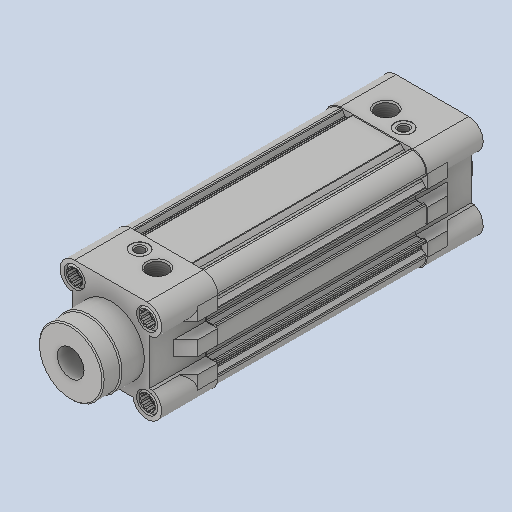
# Autodesk Inventor part: 163321 DNC-32-50---(ZR)_CPY
Saved by Autodesk Inventor 2023 (Build 270158000, 158)
## iProperties
Created: 2023-04-07
Part Number: 163321 DNC-32-50---(ZR)_CPY
Material: Generic
Catalog Web Link: www.cadenas.de
Description: DNC-(ZR)-Standard cylinder
Vendor: FESTO
Document SubType Name: Modeling
Designer: Lenovo
Manufacturer: FESTO
Mass: 206.257 g
Surface Area: 617.501 cm^2
Volume: 206.257 cm^3
Density: 1 g/cm^3
Appearance: PSOLRGB-175-175-175
Category: PARTsolutions
Company: FESTO
Title: DNC-32-50---(ZR)
Author: Cadenas PARTsolutions
Comments: Standard cylinder
PSOL_IDENT_0: {$CADENAS_DATA/23d-libs/festo/parts/d/dnc/parts/dnc_zyl.prj},223 {VTYP=3D},{NB=163321 DNC-32-50---(Z
PSOL_IDENT_1: R)},{LINA=DNC-32-50---(ZR)},{NN=DNC-(ZR)},{DATE=06.03.2020 08:57:36},{GEOMDATE=06.03.2020 08:57:36},
PSOL_IDENT_2: {VERSION=},{LINEID=10},{WBVAR=TNR,HUB,C180,Q,S2,TT,EL},{WBNUMERIC=HUB,C180,Q,S2,TT,EL}  {NB=163321 D
PSOL_IDENT_3: NC-32-50---(ZR)},{LINA=DNC-32-50---(ZR)},{KT=DUMMY},{TNR=163321},{TYP=DNC},{KDM=32},{T1=5.500},{HUB=
PSOL_IDENT_4: 50},{C180=0},{Q=0},{S2=1},{TT=0},{TTT=},{EL=0},{ZZ=0},{B=30.000},{D2=12.000},{B1=10.000},{D5=32.500}
PSOL_IDENT_5: ,{D7=M6},{D7N=6.000},{D7K=4.917},{E=45.500},{EE=G1/8},{EEN=9.728},{EEK=8.566},{EET=11.000},{J3=5.200
PSOL_IDENT_6: },{J4=6},{J5=44.500},{L2=41.600},{L3=62.800},{L4=4.000},{L5=25.100},{L6=16.000},{L7=3.300},{L8=10.00
PSOL_IDENT_7: 0},{VD=18.000},{WH=26.000},{ZB=120.000},{NA=13.700},{RE=6.000},{VL2=22.000},{C180T=},{QT=},{QN=0},{S
PSOL_IDENT_8: 2T=},{S2N=1},{ZM=97},{A1=35.000},{A2=500.000},{K1=M10},{ELT=},{ELD=13.000},{ELAV=13.900},{ELAH=12.00
PSOL_IDENT_9: 0},{ELH=10.000},{ELD2=3.000},{ELD3=1.500},{ELT1=2.000},{ELB1=6.000},{H1=57.500},{H10=7.000},{H11=0.0
PSOL_IDENT_10: 00},{MASSBASIC=0.517},{MASSHUB=0.030},{B10=6.500},{B11=7.000},{B12=10.000},{B13=11.500},{B14=2.100},
PSOL_IDENT_11: {B15=5.450},{L20=9.000},{L21=1.000},{B1ZNCM=30.000},{T2=21.000},{D100=9.500},{D101=9.000},{ANG=40.00
PSOL_IDENT_12: 0},{D102=7.400},{SW100=6.000},{L13=4.000},{V1=1.000}
NB: 163321 DNC-32-50---(ZR)
NN: DNC-(ZR)
NT: Standard cylinder
NBSYN: $TNR. $TYP.-$KDM.-$HUB.$C180T.$QT.$S2T.$TTT.$ELT.---(ZR)
LINA: DNC-32-50---(ZR)
CATALOG: Festo
TNR: 163321
TYP: DNC
KDM: 32
T1: 5.5
HUB: 50
C180: -
Q: rund
S2: normal
TT: -
EL: -
B: 30
D2: 12
B1: 10
D5: 32.5
D7: M6
D7N: 6
D7K: 4.917
E: 45.5
EE: G1/8
EEN: 9.728
EEK: 8.566
EET: 11
J3: 5.2
J4: 6
J5: 44.5
L2: 41.6
L3: 62.8
L4: 4
L5: 25.1
L6: 16
L7: 3.3
L8: 10
VD: 18
WH: 26
ZB: 120
NA: 13.7
RE: 6
VL2: 22
A1: 35
A2: 500
K1: M10
ELD: 13
ELAV: 13.9
ELAH: 12
ELH: 10
ELD2: 3
ELD3: 1.5
ELT1: 2
ELB1: 6
H1: 57.5
H10: 7
H11: 0
MASSBASIC: 0.517
MASSHUB: 0.03
B10: 6.5
B11: 7
B12: 10
B13: 11.5
B14: 2.1
B15: 5.45
L20: 9
L21: 1
B1ZNCM: 30
T2: 21
D100: 9.5
D101: 9
ANG: 40
D102: 7.4
SW100: 6
L13: 4
V1: 1
SUPPLIER: FESTO
ARTICLENO: 163321 DNC-32-50---(ZR)
BOMINFO: DNC-32-50---(ZR)
CREATOR: CADENAS GmbH
Autodesk Inventor part; units mm, degrees
sketch "Skizze_1" plane through (0, 0, 0) normal (0, 0, 1) x (1, 0, 0)
  arc A0 (-17.3, -9.8354) -> (-9.8354, -17.3) centre (-16.25, -16.25) ccw
  line L0 (-9.8354, -17.3) -> (9.8354, -17.3)
  arc A1 (9.8354, -17.3) -> (17.3, -9.8354) centre (16.25, -16.25) ccw
  line L1 (17.3, -9.8354) -> (17.3, 9.8354)
  arc A2 (17.3, 9.8354) -> (16.25, 22.75) centre (16.25, 16.25) ccw
  line L2 (16.25, 22.75) -> (-16.25, 22.75)
  arc A3 (-16.25, 22.75) -> (-17.3, 9.8354) centre (-16.25, 16.25) ccw
  line L3 (-17.3, 9.8354) -> (-17.3, -9.8354)
  constraints: 8 end point, 8 point on circle, 4 centre point
extrude "Extrusion1" add sketch "Skizze_1" against normal blind 25.1
sketch "Sketch_3" plane through (0, 0, 0) normal (1, 0, 0) x (0, 1, 0)
  line L0 (-17.3, -10.65) -> (-22.75, -16.1)
  line L1 (-22.75, -16.1) -> (-22.75, -25.1)
  line L2 (-22.75, -25.1) -> (-17.3, -25.1)
  line L3 (-17.3, -25.1) -> (-17.3, -10.65)
  constraints: 8 end point
extrude "Extrusion2" add sketch "Sketch_3" along normal mid plane 32.5
sketch "Sketch_4" plane through (0, 0, 0) normal (0, 1, 0) x (-1, 0, 0)
  line L0 (-17.3, -10.65) -> (-22.75, -16.1)
  line L1 (-22.75, -16.1) -> (-22.75, -25.1)
  line L2 (-22.75, -25.1) -> (-17.3, -25.1)
  line L3 (-17.3, -25.1) -> (-17.3, -10.65)
  constraints: 8 end point
extrude "Extrusion3" add sketch "Sketch_4" along normal mid plane 32.5
sketch "Sketch_5" plane through (0, 0, 0) normal (0, 1, 0) x (-1, 0, 0)
  line L0 (22.75, -16.1) -> (17.3, -10.65)
  line L1 (17.3, -10.65) -> (17.3, -25.1)
  line L2 (17.3, -25.1) -> (22.75, -25.1)
  line L3 (22.75, -25.1) -> (22.75, -16.1)
  constraints: 8 end point
extrude "Extrusion4" add sketch "Sketch_5" along normal mid plane 32.5
sketch "Sketch_9" plane through (0, 0, 0) normal (0, 0, 1) x (1, 0, 0)
  line L0 (-27.75, 10.25) -> (-27.75, -27.75)
  line L1 (-27.75, -27.75) -> (27.75, -27.75)
  line L2 (27.75, -27.75) -> (27.75, 10.25)
  line L3 (27.75, 10.25) -> (17.3, 10.25)
  line L4 (17.3, 10.25) -> (17.3, 3.25)
  line L5 (17.3, 3.25) -> (25.75, 3.25)
  line L6 (25.75, 3.25) -> (25.75, -3.25)
  line L7 (25.75, -3.25) -> (17.3, -3.25)
  line L8 (17.3, -3.25) -> (17.3, -10.25)
  line L9 (17.3, -10.25) -> (25.75, -10.25)
  line L10 (25.75, -10.25) -> (25.75, -25.75)
  line L11 (25.75, -25.75) -> (10.25, -25.75)
  line L12 (10.25, -25.75) -> (10.25, -17.3)
  line L13 (10.25, -17.3) -> (3.25, -17.3)
  line L14 (3.25, -17.3) -> (3.25, -25.75)
  line L15 (3.25, -25.75) -> (-3.25, -25.75)
  line L16 (-3.25, -25.75) -> (-3.25, -17.3)
  line L17 (-3.25, -17.3) -> (-10.25, -17.3)
  line L18 (-10.25, -17.3) -> (-10.25, -25.75)
  line L19 (-10.25, -25.75) -> (-25.75, -25.75)
  line L20 (-25.75, -25.75) -> (-25.75, -10.25)
  line L21 (-25.75, -10.25) -> (-17.3, -10.25)
  line L22 (-17.3, -10.25) -> (-17.3, -3.25)
  line L23 (-17.3, -3.25) -> (-25.75, -3.25)
  line L24 (-25.75, -3.25) -> (-25.75, 3.25)
  line L25 (-25.75, 3.25) -> (-17.3, 3.25)
  line L26 (-17.3, 3.25) -> (-17.3, 10.25)
  line L27 (-17.3, 10.25) -> (-27.75, 10.25)
  constraints: 56 end point
extrude "Extrusion5" cut sketch "Sketch_9" against normal blind 25.1
sketch "Skizze_2" plane through (0, 0, -25.1) normal (0, 0, 1) x (1, 0, 0)
  arc A0 (-22.25, -16.25) -> (-16.25, -22.25) centre (-16.25, -16.25) ccw
  line L0 (-16.25, -22.25) -> (-15.4099, -22.25)
  arc A1 (-15.4099, -22.25) -> (-15.0635, -22.05) centre (-15.4099, -21.85) ccw
  line L1 (-15.0635, -22.05) -> (-14.082, -20.35)
  arc A2 (-13.7356, -20.15) -> (-14.082, -20.35) centre (-13.7356, -20.55) ccw
  line L2 (-13.7356, -20.15) -> (-13.4713, -20.15)
  arc A3 (-12.4107, -20.5893) -> (-13.4713, -20.15) centre (-13.4713, -21.65) ccw
  line L3 (-12.4107, -20.5893) -> (-10.8672, -22.1328)
  arc A4 (-10.8672, -22.1328) -> (-10.5843, -22.25) centre (-10.5843, -21.85) ccw
  line L4 (-10.5843, -22.25) -> (-9.85, -22.25)
  arc A5 (-9.85, -22.25) -> (-9.45, -21.85) centre (-9.85, -21.85) ccw
  line L5 (-9.45, -21.85) -> (-9.45, -21.15)
  arc A6 (-9.45, -21.15) -> (-9.65, -20.95) centre (-9.65, -21.15) ccw
  line L6 (-9.65, -20.95) -> (-9.9, -20.95)
  arc A7 (-10.1, -20.75) -> (-9.9, -20.95) centre (-9.9, -20.75) ccw
  line L7 (-10.1, -20.75) -> (-10.1, -18.05)
  arc A8 (-9.7, -17.65) -> (-10.1, -18.05) centre (-9.7, -18.05) ccw
  line L8 (-9.7, -17.65) -> (-4, -17.65)
  arc A9 (-3.6, -18.05) -> (-4, -17.65) centre (-4, -18.05) ccw
  line L9 (-3.6, -18.05) -> (-3.6, -20.75)
  arc A10 (-3.8, -20.95) -> (-3.6, -20.75) centre (-3.8, -20.75) ccw
  line L10 (-3.8, -20.95) -> (-4.05, -20.95)
  arc A11 (-4.05, -20.95) -> (-4.25, -21.15) centre (-4.05, -21.15) ccw
  line L11 (-4.25, -21.15) -> (-4.25, -21.85)
  arc A12 (-4.25, -21.85) -> (-3.85, -22.25) centre (-3.85, -21.85) ccw
  line L12 (-3.85, -22.25) -> (3.85, -22.25)
  arc A13 (3.85, -22.25) -> (4.25, -21.85) centre (3.85, -21.85) ccw
  line L13 (4.25, -21.85) -> (4.25, -21.15)
  arc A14 (4.25, -21.15) -> (4.05, -20.95) centre (4.05, -21.15) ccw
  line L14 (4.05, -20.95) -> (3.8, -20.95)
  arc A15 (3.6, -20.75) -> (3.8, -20.95) centre (3.8, -20.75) ccw
  line L15 (3.6, -20.75) -> (3.6, -18.05)
  arc A16 (4, -17.65) -> (3.6, -18.05) centre (4, -18.05) ccw
  line L16 (4, -17.65) -> (9.7, -17.65)
  arc A17 (10.1, -18.05) -> (9.7, -17.65) centre (9.7, -18.05) ccw
  line L17 (10.1, -18.05) -> (10.1, -20.75)
  arc A18 (9.9, -20.95) -> (10.1, -20.75) centre (9.9, -20.75) ccw
  line L18 (9.9, -20.95) -> (9.65, -20.95)
  arc A19 (9.65, -20.95) -> (9.45, -21.15) centre (9.65, -21.15) ccw
  line L19 (9.45, -21.15) -> (9.45, -21.85)
  arc A20 (9.45, -21.85) -> (9.85, -22.25) centre (9.85, -21.85) ccw
  line L20 (9.85, -22.25) -> (10.5843, -22.25)
  arc A21 (10.5843, -22.25) -> (10.8672, -22.1328) centre (10.5843, -21.85) ccw
  line L21 (10.8672, -22.1328) -> (12.4107, -20.5893)
  arc A22 (13.4713, -20.15) -> (12.4107, -20.5893) centre (13.4713, -21.65) ccw
  line L22 (13.4713, -20.15) -> (13.7356, -20.15)
  arc A23 (14.082, -20.35) -> (13.7356, -20.15) centre (13.7356, -20.55) ccw
  line L23 (14.082, -20.35) -> (15.0635, -22.05)
  arc A24 (15.0635, -22.05) -> (15.4099, -22.25) centre (15.4099, -21.85) ccw
  line L24 (15.4099, -22.25) -> (16.25, -22.25)
  arc A25 (16.25, -22.25) -> (22.25, -16.25) centre (16.25, -16.25) ccw
  line L25 (22.25, -16.25) -> (22.25, -15.4099)
  arc A26 (22.25, -15.4099) -> (22.05, -15.0635) centre (21.85, -15.4099) ccw
  line L26 (22.05, -15.0635) -> (20.35, -14.082)
  arc A27 (20.15, -13.7356) -> (20.35, -14.082) centre (20.55, -13.7356) ccw
  line L27 (20.15, -13.7356) -> (20.15, -13.4713)
  arc A28 (20.5893, -12.4107) -> (20.15, -13.4713) centre (21.65, -13.4713) ccw
  line L28 (20.5893, -12.4107) -> (22.1328, -10.8672)
  arc A29 (22.1328, -10.8672) -> (22.25, -10.5843) centre (21.85, -10.5843) ccw
  line L29 (22.25, -10.5843) -> (22.25, -9.85)
  arc A30 (22.25, -9.85) -> (21.85, -9.45) centre (21.85, -9.85) ccw
  line L30 (21.85, -9.45) -> (21.15, -9.45)
  arc A31 (21.15, -9.45) -> (20.95, -9.65) centre (21.15, -9.65) ccw
  line L31 (20.95, -9.65) -> (20.95, -9.9)
  arc A32 (20.75, -10.1) -> (20.95, -9.9) centre (20.75, -9.9) ccw
  line L32 (20.75, -10.1) -> (18.05, -10.1)
  arc A33 (17.65, -9.7) -> (18.05, -10.1) centre (18.05, -9.7) ccw
  line L33 (17.65, -9.7) -> (17.65, -4)
  arc A34 (18.05, -3.6) -> (17.65, -4) centre (18.05, -4) ccw
  line L34 (18.05, -3.6) -> (20.75, -3.6)
  arc A35 (20.95, -3.8) -> (20.75, -3.6) centre (20.75, -3.8) ccw
  line L35 (20.95, -3.8) -> (20.95, -4.05)
  arc A36 (20.95, -4.05) -> (21.15, -4.25) centre (21.15, -4.05) ccw
  line L36 (21.15, -4.25) -> (21.85, -4.25)
  arc A37 (21.85, -4.25) -> (22.25, -3.85) centre (21.85, -3.85) ccw
  line L37 (22.25, -3.85) -> (22.25, 3.85)
  arc A38 (22.25, 3.85) -> (21.85, 4.25) centre (21.85, 3.85) ccw
  line L38 (21.85, 4.25) -> (21.15, 4.25)
  arc A39 (21.15, 4.25) -> (20.95, 4.05) centre (21.15, 4.05) ccw
  line L39 (20.95, 4.05) -> (20.95, 3.8)
  arc A40 (20.75, 3.6) -> (20.95, 3.8) centre (20.75, 3.8) ccw
  line L40 (20.75, 3.6) -> (18.05, 3.6)
  arc A41 (17.65, 4) -> (18.05, 3.6) centre (18.05, 4) ccw
  line L41 (17.65, 4) -> (17.65, 9.7)
  arc A42 (18.05, 10.1) -> (17.65, 9.7) centre (18.05, 9.7) ccw
  line L42 (18.05, 10.1) -> (20.75, 10.1)
  arc A43 (20.95, 9.9) -> (20.75, 10.1) centre (20.75, 9.9) ccw
  line L43 (20.95, 9.9) -> (20.95, 9.65)
  arc A44 (20.95, 9.65) -> (21.15, 9.45) centre (21.15, 9.65) ccw
  line L44 (21.15, 9.45) -> (21.85, 9.45)
  arc A45 (21.85, 9.45) -> (22.25, 9.85) centre (21.85, 9.85) ccw
  line L45 (22.25, 9.85) -> (22.25, 10.5843)
  arc A46 (22.25, 10.5843) -> (22.1328, 10.8672) centre (21.85, 10.5843) ccw
  line L46 (22.1328, 10.8672) -> (20.5893, 12.4107)
  arc A47 (20.15, 13.4713) -> (20.5893, 12.4107) centre (21.65, 13.4713) ccw
  line L47 (20.15, 13.4713) -> (20.15, 13.7356)
  arc A48 (20.35, 14.082) -> (20.15, 13.7356) centre (20.55, 13.7356) ccw
  line L48 (20.35, 14.082) -> (22.05, 15.0635)
  arc A49 (22.05, 15.0635) -> (22.25, 15.4099) centre (21.85, 15.4099) ccw
  line L49 (22.25, 15.4099) -> (22.25, 16.25)
  arc A50 (22.25, 16.25) -> (16.25, 22.25) centre (16.25, 16.25) ccw
  line L50 (16.25, 22.25) -> (15.4099, 22.25)
  arc A51 (15.4099, 22.25) -> (15.0635, 22.05) centre (15.4099, 21.85) ccw
  line L51 (15.0635, 22.05) -> (14.082, 20.35)
  arc A52 (13.7356, 20.15) -> (14.082, 20.35) centre (13.7356, 20.55) ccw
  line L52 (13.7356, 20.15) -> (13.4713, 20.15)
  arc A53 (12.4107, 20.5893) -> (13.4713, 20.15) centre (13.4713, 21.65) ccw
  line L53 (12.4107, 20.5893) -> (10.8672, 22.1328)
  arc A54 (10.8672, 22.1328) -> (10.5843, 22.25) centre (10.5843, 21.85) ccw
  line L54 (10.5843, 22.25) -> (-10.5843, 22.25)
  arc A55 (-10.5843, 22.25) -> (-10.8672, 22.1328) centre (-10.5843, 21.85) ccw
  line L55 (-10.8672, 22.1328) -> (-12.4107, 20.5893)
  arc A56 (-13.4713, 20.15) -> (-12.4107, 20.5893) centre (-13.4713, 21.65) ccw
  line L56 (-13.4713, 20.15) -> (-13.7356, 20.15)
  arc A57 (-14.082, 20.35) -> (-13.7356, 20.15) centre (-13.7356, 20.55) ccw
  line L57 (-14.082, 20.35) -> (-15.0635, 22.05)
  arc A58 (-15.0635, 22.05) -> (-15.4099, 22.25) centre (-15.4099, 21.85) ccw
  line L58 (-15.4099, 22.25) -> (-16.25, 22.25)
  arc A59 (-16.25, 22.25) -> (-22.25, 16.25) centre (-16.25, 16.25) ccw
  line L59 (-22.25, 16.25) -> (-22.25, 15.4099)
  arc A60 (-22.25, 15.4099) -> (-22.05, 15.0635) centre (-21.85, 15.4099) ccw
  line L60 (-22.05, 15.0635) -> (-20.35, 14.082)
  arc A61 (-20.15, 13.7356) -> (-20.35, 14.082) centre (-20.55, 13.7356) ccw
  line L61 (-20.15, 13.7356) -> (-20.15, 13.4713)
  arc A62 (-20.5893, 12.4107) -> (-20.15, 13.4713) centre (-21.65, 13.4713) ccw
  line L62 (-20.5893, 12.4107) -> (-22.1328, 10.8672)
  arc A63 (-22.1328, 10.8672) -> (-22.25, 10.5843) centre (-21.85, 10.5843) ccw
  line L63 (-22.25, 10.5843) -> (-22.25, 9.85)
  arc A64 (-22.25, 9.85) -> (-21.85, 9.45) centre (-21.85, 9.85) ccw
  line L64 (-21.85, 9.45) -> (-21.15, 9.45)
  arc A65 (-21.15, 9.45) -> (-20.95, 9.65) centre (-21.15, 9.65) ccw
  line L65 (-20.95, 9.65) -> (-20.95, 9.9)
  arc A66 (-20.75, 10.1) -> (-20.95, 9.9) centre (-20.75, 9.9) ccw
  line L66 (-20.75, 10.1) -> (-18.05, 10.1)
  arc A67 (-17.65, 9.7) -> (-18.05, 10.1) centre (-18.05, 9.7) ccw
  line L67 (-17.65, 9.7) -> (-17.65, 4)
  arc A68 (-18.05, 3.6) -> (-17.65, 4) centre (-18.05, 4) ccw
  line L68 (-18.05, 3.6) -> (-20.75, 3.6)
  arc A69 (-20.95, 3.8) -> (-20.75, 3.6) centre (-20.75, 3.8) ccw
  line L69 (-20.95, 3.8) -> (-20.95, 4.05)
  arc A70 (-20.95, 4.05) -> (-21.15, 4.25) centre (-21.15, 4.05) ccw
  line L70 (-21.15, 4.25) -> (-21.85, 4.25)
  arc A71 (-21.85, 4.25) -> (-22.25, 3.85) centre (-21.85, 3.85) ccw
  line L71 (-22.25, 3.85) -> (-22.25, -3.85)
  arc A72 (-22.25, -3.85) -> (-21.85, -4.25) centre (-21.85, -3.85) ccw
  line L72 (-21.85, -4.25) -> (-21.15, -4.25)
  arc A73 (-21.15, -4.25) -> (-20.95, -4.05) centre (-21.15, -4.05) ccw
  line L73 (-20.95, -4.05) -> (-20.95, -3.8)
  arc A74 (-20.75, -3.6) -> (-20.95, -3.8) centre (-20.75, -3.8) ccw
  line L74 (-20.75, -3.6) -> (-18.05, -3.6)
  arc A75 (-17.65, -4) -> (-18.05, -3.6) centre (-18.05, -4) ccw
  line L75 (-17.65, -4) -> (-17.65, -9.7)
  arc A76 (-18.05, -10.1) -> (-17.65, -9.7) centre (-18.05, -9.7) ccw
  line L76 (-18.05, -10.1) -> (-20.75, -10.1)
  arc A77 (-20.95, -9.9) -> (-20.75, -10.1) centre (-20.75, -9.9) ccw
  line L77 (-20.95, -9.9) -> (-20.95, -9.65)
  arc A78 (-20.95, -9.65) -> (-21.15, -9.45) centre (-21.15, -9.65) ccw
  line L78 (-21.15, -9.45) -> (-21.85, -9.45)
  arc A79 (-21.85, -9.45) -> (-22.25, -9.85) centre (-21.85, -9.85) ccw
  line L79 (-22.25, -9.85) -> (-22.25, -10.5843)
  arc A80 (-22.25, -10.5843) -> (-22.1328, -10.8672) centre (-21.85, -10.5843) ccw
  line L80 (-22.1328, -10.8672) -> (-20.5893, -12.4107)
  arc A81 (-20.15, -13.4713) -> (-20.5893, -12.4107) centre (-21.65, -13.4713) ccw
  line L81 (-20.15, -13.4713) -> (-20.15, -13.7356)
  arc A82 (-20.35, -14.082) -> (-20.15, -13.7356) centre (-20.55, -13.7356) ccw
  line L82 (-20.35, -14.082) -> (-22.05, -15.0635)
  arc A83 (-22.05, -15.0635) -> (-22.25, -15.4099) centre (-21.85, -15.4099) ccw
  line L83 (-22.25, -15.4099) -> (-22.25, -16.25)
  constraints: 168 end point, 168 point on circle, 84 centre point
extrude "Extrusion6" add sketch "Skizze_2" against normal blind 93.8
sketch "Skizze_3" plane through (0, 0, -118.9) normal (0, 0, 1) x (1, 0, 0)
  arc A0 (-17.3, -9.8354) -> (-9.8354, -17.3) centre (-16.25, -16.25) ccw
  line L0 (-9.8354, -17.3) -> (9.8354, -17.3)
  arc A1 (9.8354, -17.3) -> (17.3, -9.8354) centre (16.25, -16.25) ccw
  line L1 (17.3, -9.8354) -> (17.3, 9.8354)
  arc A2 (17.3, 9.8354) -> (16.25, 22.75) centre (16.25, 16.25) ccw
  line L2 (16.25, 22.75) -> (-16.25, 22.75)
  arc A3 (-16.25, 22.75) -> (-17.3, 9.8354) centre (-16.25, 16.25) ccw
  line L3 (-17.3, 9.8354) -> (-17.3, -9.8354)
  constraints: 8 end point, 8 point on circle, 4 centre point
extrude "Extrusion7" add sketch "Skizze_3" against normal blind 25.1
sketch "Sketch_6" plane through (0, 0, 0) normal (1, 0, 0) x (0, 1, 0)
  line L0 (-17.3, -118.9) -> (-22.75, -118.9)
  line L1 (-22.75, -118.9) -> (-22.75, -127.9)
  line L2 (-22.75, -127.9) -> (-17.3, -133.35)
  line L3 (-17.3, -133.35) -> (-17.3, -118.9)
  constraints: 8 end point
extrude "Extrusion8" add sketch "Sketch_6" along normal mid plane 32.5
sketch "Sketch_7" plane through (0, 0, 0) normal (0, 1, 0) x (-1, 0, 0)
  line L0 (-17.3, -133.35) -> (-17.3, -118.9)
  line L1 (-17.3, -118.9) -> (-22.75, -118.9)
  line L2 (-22.75, -118.9) -> (-22.75, -127.9)
  line L3 (-22.75, -127.9) -> (-17.3, -133.35)
  constraints: 8 end point
extrude "Extrusion9" add sketch "Sketch_7" along normal mid plane 32.5
sketch "Sketch_8" plane through (0, 0, 0) normal (0, 1, 0) x (-1, 0, 0)
  line L0 (22.75, -127.9) -> (22.75, -118.9)
  line L1 (22.75, -118.9) -> (17.3, -118.9)
  line L2 (17.3, -118.9) -> (17.3, -133.35)
  line L3 (17.3, -133.35) -> (22.75, -127.9)
  constraints: 8 end point
extrude "Extrusion10" add sketch "Sketch_8" along normal mid plane 32.5
sketch "Sketch_10" plane through (0, 0, -118.9) normal (0, 0, 1) x (1, 0, 0)
  line L0 (-27.75, 10.25) -> (-27.75, -27.75)
  line L1 (-27.75, -27.75) -> (27.75, -27.75)
  line L2 (27.75, -27.75) -> (27.75, 10.25)
  line L3 (27.75, 10.25) -> (17.3, 10.25)
  line L4 (17.3, 10.25) -> (17.3, 3.25)
  line L5 (17.3, 3.25) -> (25.75, 3.25)
  line L6 (25.75, 3.25) -> (25.75, -3.25)
  line L7 (25.75, -3.25) -> (17.3, -3.25)
  line L8 (17.3, -3.25) -> (17.3, -10.25)
  line L9 (17.3, -10.25) -> (25.75, -10.25)
  line L10 (25.75, -10.25) -> (25.75, -25.75)
  line L11 (25.75, -25.75) -> (10.25, -25.75)
  line L12 (10.25, -25.75) -> (10.25, -17.3)
  line L13 (10.25, -17.3) -> (3.25, -17.3)
  line L14 (3.25, -17.3) -> (3.25, -25.75)
  line L15 (3.25, -25.75) -> (-3.25, -25.75)
  line L16 (-3.25, -25.75) -> (-3.25, -17.3)
  line L17 (-3.25, -17.3) -> (-10.25, -17.3)
  line L18 (-10.25, -17.3) -> (-10.25, -25.75)
  line L19 (-10.25, -25.75) -> (-25.75, -25.75)
  line L20 (-25.75, -25.75) -> (-25.75, -10.25)
  line L21 (-25.75, -10.25) -> (-17.3, -10.25)
  line L22 (-17.3, -10.25) -> (-17.3, -3.25)
  line L23 (-17.3, -3.25) -> (-25.75, -3.25)
  line L24 (-25.75, -3.25) -> (-25.75, 3.25)
  line L25 (-25.75, 3.25) -> (-17.3, 3.25)
  line L26 (-17.3, 3.25) -> (-17.3, 10.25)
  line L27 (-17.3, 10.25) -> (-27.75, 10.25)
  constraints: 56 end point
extrude "Extrusion11" cut sketch "Sketch_10" against normal blind 25.1
sketch "Sketch_14" plane through (16.25, 0, 0) normal (1, 0, 0) x (0, 0, -1)
  line L0 (21, 16.25) -> (0, 16.25)
  line L1 (0, 16.25) -> (0, 21)
  line L2 (0, 21) -> (21, 21)
  line L3 (21, 21) -> (21, 16.25)
  line L4 (21, 16.25) -> (0, 16.25)
  constraints: 10 end point
revolve "Revolution1" cut sketch "Sketch_14" angle 360 about axis through (16.25, 16.25, -21) along (0, 0, -1)
pattern_linear "Rectangular Pattern1" count 2 spacing 32.5 along (-1, 0, 0) count 2 spacing 32.5 along (0, -1, 0) of "Revolution1"
sketch "Sketch_15" plane through (16.25, 0, 0) normal (1, 0, 0) x (0, 0, -1)
  line L0 (21, 16.25) -> (0, 16.25)
  line L1 (0, 16.25) -> (0, 19.9109)
  line L2 (0, 19.9109) -> (1, 20.75)
  line L3 (1, 20.75) -> (21, 20.75)
  line L4 (21, 20.75) -> (21, 16.25)
  line L5 (21, 16.25) -> (0, 16.25)
  constraints: 12 end point
revolve "Revolution2" add sketch "Sketch_15" angle 360 about axis through (16.25, 16.25, -21) along (0, 0, -1)
pattern_linear "Rectangular Pattern2" count 2 spacing 32.5 along (-1, 0, 0) count 2 spacing 32.5 along (0, -1, 0) of "Revolution2"
sketch "Skizze_8" plane through (16.25, 0, 0) normal (1, 0, 0) x (0, 0, -1)
  line L0 (21.3333, 16.25) -> (0, 16.25)
  line L1 (0, 16.25) -> (0, 19.95)
  line L2 (0, 19.95) -> (0.4041, 19.25)
  line L3 (0.4041, 19.25) -> (5.5, 19.25)
  line L4 (5.5, 19.25) -> (6.0415, 18.7085)
  line L5 (6.0415, 18.7085) -> (19.9139, 18.7085)
  line L6 (19.9139, 18.7085) -> (21.3333, 16.25)
  line L7 (21.3333, 16.25) -> (0, 16.25)
  constraints: 16 end point
revolve "Revolution3" cut sketch "Skizze_8" angle 360 about axis through (16.25, 16.25, -21.3333) along (0, 0, -1)
thread "Thread1" size "M6x1" class "6H" standard "ISO Metric profile" length 9.9585
pattern_linear "Rectangular Pattern3" count 2 spacing 32.5 along (-1, 0, 0) count 2 spacing 32.5 along (0, -1, 0) of "Revolution3"
sketch "Sketch_19" plane through (0, 0, 0) normal (0, 0, 1) x (1, 0, 0)
  line L0 (12.7859, 16.25) -> (13.25, 15.4462)
  line L1 (13.25, 15.4462) -> (13.25, 14.5179)
  line L2 (13.25, 14.5179) -> (14.0538, 14.0538)
  line L3 (14.0538, 14.0538) -> (14.5179, 13.25)
  line L4 (14.5179, 13.25) -> (15.4462, 13.25)
  line L5 (15.4462, 13.25) -> (16.25, 12.7859)
  line L6 (16.25, 12.7859) -> (17.0538, 13.25)
  line L7 (17.0538, 13.25) -> (17.9821, 13.25)
  line L8 (17.9821, 13.25) -> (18.4462, 14.0538)
  line L9 (18.4462, 14.0538) -> (19.25, 14.5179)
  line L10 (19.25, 14.5179) -> (19.25, 15.4462)
  line L11 (19.25, 15.4462) -> (19.7141, 16.25)
  line L12 (19.7141, 16.25) -> (19.25, 17.0538)
  line L13 (19.25, 17.0538) -> (19.25, 17.9821)
  line L14 (19.25, 17.9821) -> (18.4462, 18.4462)
  line L15 (18.4462, 18.4462) -> (17.9821, 19.25)
  line L16 (17.9821, 19.25) -> (17.0538, 19.25)
  line L17 (17.0538, 19.25) -> (16.25, 19.7141)
  line L18 (16.25, 19.7141) -> (15.4462, 19.25)
  line L19 (15.4462, 19.25) -> (14.5179, 19.25)
  line L20 (14.5179, 19.25) -> (14.0538, 18.4462)
  line L21 (14.0538, 18.4462) -> (13.25, 17.9821)
  line L22 (13.25, 17.9821) -> (13.25, 17.0538)
  line L23 (13.25, 17.0538) -> (12.7859, 16.25)
  constraints: 48 end point
extrude "Extrusion12" cut sketch "Sketch_19" against normal blind 4
pattern_linear "Rectangular Pattern4" count 2 spacing 32.5 along (-1, 0, 0) count 2 spacing 32.5 along (0, -1, 0) of "Extrusion12"
sketch "Sketch16" plane through (0, 0, -144) normal (0, 0, -1) x (-1, 0, 0)
  point P0 (-16.25, 16.25)
hole "Hole1" at (16.25, 16.25, -144) direction (0, 0, 1) diameter 9.5 depth 21
pattern_linear "Rectangular Pattern5" count 2 spacing 32.5 along (-1, 0, 0) count 2 spacing 32.5 along (0, -1, 0) of "Hole1"
sketch "Sketch_23" plane through (16.25, 0, 0) normal (1, 0, 0) x (0, 0, -1)
  line L0 (144, 16.25) -> (123, 16.25)
  line L1 (123, 16.25) -> (123, 20.75)
  line L2 (123, 20.75) -> (143, 20.75)
  line L3 (143, 20.75) -> (144, 19.9109)
  line L4 (144, 19.9109) -> (144, 16.25)
  line L5 (144, 16.25) -> (123, 16.25)
  constraints: 12 end point
revolve "Revolution4" add sketch "Sketch_23" angle 360 about axis through (16.25, 16.25, -144) along (0, 0, -1)
pattern_linear "Rectangular Pattern6" count 2 spacing 32.5 along (-1, 0, 0) count 2 spacing 32.5 along (0, -1, 0) of "Revolution4"
sketch "Sketch_25" plane through (16.25, 0, 0) normal (1, 0, 0) x (0, 0, -1)
  line L0 (144, 16.25) -> (122.6667, 16.25)
  line L1 (122.6667, 16.25) -> (124.0861, 18.7085)
  line L2 (124.0861, 18.7085) -> (137.9585, 18.7085)
  line L3 (137.9585, 18.7085) -> (138.5, 19.25)
  line L4 (138.5, 19.25) -> (143.5959, 19.25)
  line L5 (143.5959, 19.25) -> (144, 19.95)
  line L6 (144, 19.95) -> (144, 16.25)
  line L7 (144, 16.25) -> (122.6667, 16.25)
  constraints: 16 end point
revolve "Revolution5" cut sketch "Sketch_25" angle 360 about axis through (16.25, 16.25, -144) along (0, 0, -1)
thread "Thread2" size "M6x1" class "6H" standard "ISO Metric profile" length 9.9585
pattern_linear "Rectangular Pattern7" count 2 spacing 32.5 along (-1, 0, 0) count 2 spacing 32.5 along (0, -1, 0) of "Revolution5"
sketch "Sketch_27" plane through (0, 0, -144) normal (0, 0, 1) x (1, 0, 0)
  line L0 (12.7859, 16.25) -> (13.25, 15.4462)
  line L1 (13.25, 15.4462) -> (13.25, 14.5179)
  line L2 (13.25, 14.5179) -> (14.0538, 14.0538)
  line L3 (14.0538, 14.0538) -> (14.5179, 13.25)
  line L4 (14.5179, 13.25) -> (15.4462, 13.25)
  line L5 (15.4462, 13.25) -> (16.25, 12.7859)
  line L6 (16.25, 12.7859) -> (17.0538, 13.25)
  line L7 (17.0538, 13.25) -> (17.9821, 13.25)
  line L8 (17.9821, 13.25) -> (18.4462, 14.0538)
  line L9 (18.4462, 14.0538) -> (19.25, 14.5179)
  line L10 (19.25, 14.5179) -> (19.25, 15.4462)
  line L11 (19.25, 15.4462) -> (19.7141, 16.25)
  line L12 (19.7141, 16.25) -> (19.25, 17.0538)
  line L13 (19.25, 17.0538) -> (19.25, 17.9821)
  line L14 (19.25, 17.9821) -> (18.4462, 18.4462)
  line L15 (18.4462, 18.4462) -> (17.9821, 19.25)
  line L16 (17.9821, 19.25) -> (17.0538, 19.25)
  line L17 (17.0538, 19.25) -> (16.25, 19.7141)
  line L18 (16.25, 19.7141) -> (15.4462, 19.25)
  line L19 (15.4462, 19.25) -> (14.5179, 19.25)
  line L20 (14.5179, 19.25) -> (14.0538, 18.4462)
  line L21 (14.0538, 18.4462) -> (13.25, 17.9821)
  line L22 (13.25, 17.9821) -> (13.25, 17.0538)
  line L23 (13.25, 17.0538) -> (12.7859, 16.25)
  constraints: 48 end point
extrude "Extrusion13" cut sketch "Sketch_27" along normal blind 4
pattern_linear "Rectangular Pattern8" count 2 spacing 32.5 along (-1, 0, 0) count 2 spacing 32.5 along (0, -1, 0) of "Extrusion13"
sketch "Skizze_13" plane through (0, 0, 0) normal (1, 0, 0) x (0, 1, 0)
  line L0 (0, 0) -> (0, 18)
  line L1 (0, 18) -> (14, 18)
  line L2 (14, 18) -> (14.5, 17.5)
  line L3 (14.5, 17.5) -> (14.5, 10.5)
  line L4 (14.5, 10.5) -> (15, 10)
  line L5 (15, 10) -> (15, 0)
  line L6 (15, 0) -> (0, 0)
  line L7 (0, 0) -> (0, 18)
  constraints: 16 end point
revolve "Revolution6" add sketch "Skizze_13" angle 360 about axis through (0, 0, 0) along (0, 0, -1)
sketch "Sketch21" plane through (-16.25, 22.75, 0) normal (0, 1, 0) x (1, 0, 0)
  point P0 (21.45, 15.6)
hole "Hole2" at (5.2, 22.75, -15.6) direction (0, -1, 0) diameter 8.566 depth 11 countersink diameter 9.728 countersink angle 90 thread size "G9.728x0.907" designation "G 1/8" standard "ISO Pipe Threads"
sketch "Sketch_49" plane through (0, 0, -18.9) normal (0, 0, 1) x (1, 0, 0)
  line L0 (-6, 20.1167) -> (-6, 23.65)
  line L1 (-6, 23.65) -> (-2, 23.65)
  line L2 (-2, 23.65) -> (-2, 22.15)
  line L3 (-2, 22.15) -> (-2.0882, 22.65)
  line L4 (-2.0882, 22.65) -> (-3.5, 22.65)
  line L5 (-3.5, 22.65) -> (-3.933, 22.217)
  line L6 (-3.933, 22.217) -> (-3.933, 19.6167)
  line L7 (-3.933, 19.6167) -> (-4.433, 20.1167)
  line L8 (-4.433, 20.1167) -> (-6, 20.1167)
  line L9 (-6, 20.1167) -> (-6, 23.65)
  constraints: 20 end point
revolve "Revolution7" cut sketch "Sketch_49" angle 360 about axis through (-6, 20.1167, -18.9) along (0, -1, 0)
thread "Thread3" size "M5x0.8" class "6H" standard "ISO Metric profile" full length
sketch "Sketch_50" plane through (-6, 20.1167, -18.9) normal (0, 1, 0) x (1, 0, 0)
  line L0 (-0.25, -2) -> (0.25, -2)
  line L1 (0.25, -2) -> (0.25, 2)
  line L2 (0.25, 2) -> (-0.25, 2)
  line L3 (-0.25, 2) -> (-0.25, -2)
  constraints: 8 end point
extrude "Extrusion14" cut sketch "Sketch_50" against normal blind 1.5
sketch "Sketch24" plane through (-16.25, 22.75, -118.9) normal (0, 1, 0) x (1, 0, 0)
  point P0 (11.05, 9.5)
hole "Hole3" at (-5.2, 22.75, -128.4) direction (0, -1, 0) diameter 8.566 depth 11 countersink diameter 9.728 countersink angle 90 thread size "G9.728x0.907" designation "G 1/8" standard "ISO Pipe Threads"
sketch "Sketch_51" plane through (0, 0, -125.1) normal (0, 0, 1) x (1, 0, 0)
  line L0 (6, 23.65) -> (6, 20.1167)
  line L1 (6, 20.1167) -> (4.433, 20.1167)
  line L2 (4.433, 20.1167) -> (3.933, 19.6167)
  line L3 (3.933, 19.6167) -> (3.933, 22.217)
  line L4 (3.933, 22.217) -> (3.5, 22.65)
  line L5 (3.5, 22.65) -> (2.0882, 22.65)
  line L6 (2.0882, 22.65) -> (2, 22.15)
  line L7 (2, 22.15) -> (2, 23.65)
  line L8 (2, 23.65) -> (6, 23.65)
  line L9 (6, 23.65) -> (6, 20.1167)
  constraints: 20 end point
revolve "Revolution8" cut sketch "Sketch_51" angle 360 about axis through (6, 23.65, -125.1) along (0, 1, 0)
thread "Thread4" size "M5x0.8" class "6H" standard "ISO Metric profile" full length
sketch "Sketch_52" plane through (6, 20.1167, -125.1) normal (0, 1, 0) x (-1, 0, 0)
  line L0 (-0.25, -2) -> (0.25, -2)
  line L1 (0.25, -2) -> (0.25, 2)
  line L2 (0.25, 2) -> (-0.25, 2)
  line L3 (-0.25, 2) -> (-0.25, -2)
  constraints: 8 end point
extrude "Extrusion15" cut sketch "Sketch_52" against normal blind 1.5
sketch "Skizze_17" plane through (0, 0, 0) normal (1, 0, 0) x (0, 1, 0)
  line L0 (0, -148) -> (0, -144)
  line L1 (0, -144) -> (15, -144)
  line L2 (15, -144) -> (15, -147)
  line L3 (15, -147) -> (14, -148)
  line L4 (14, -148) -> (0, -148)
  line L5 (0, -148) -> (0, -144)
  constraints: 12 end point
revolve "Revolution9" add sketch "Skizze_17" angle 360 about axis through (0, 0, -148) along (0, 0, -1)
sketch "Sketch28" plane through (0, 0, 18) normal (0, 0, 1) x (1, 0, 0)
  point P0 (0, 0)
hole "Hole4" at (0, 0, 18) direction (0, 0, -1) diameter 12 depth 64.0333
sketch "Skizze_19" plane through (0, 0, 0) normal (1, 0, 0) x (0, 1, 0)
  line L0 (0, -97) -> (0, -38)
  line L1 (0, -38) -> (3, -38)
  line L2 (3, -38) -> (3, -41)
  line L3 (3, -41) -> (16, -41)
  line L4 (16, -41) -> (16, -97)
  line L5 (16, -97) -> (0, -97)
  line L6 (0, -97) -> (0, -38)
  constraints: 14 end point
revolve "Revolution10" cut sketch "Skizze_19" angle 360 about axis through (0, 0, -97) along (0, 0, -1)
ref_plane "CP_hinten_5_XY" through (16.25, 16.25, -144) normal (0, 0, 1) x (1, 0, 0)
ref_plane "CP_hinten_5_YZ" through (16.25, 16.25, -144) normal (1, 0, 0) x (0, 1, 0)
ref_plane "CP_hinten_5_ZX" through (16.25, 16.25, -144) normal (0, 1, 0) x (0, 0, 1)
ref_plane "CP_hinten_6_XY" through (16.25, -16.25, -144) normal (0, 0, 1) x (1, 0, 0)
ref_plane "CP_hinten_6_YZ" through (16.25, -16.25, -144) normal (1, 0, 0) x (0, 1, 0)
ref_plane "CP_hinten_6_ZX" through (16.25, -16.25, -144) normal (0, 1, 0) x (0, 0, 1)
ref_plane "CP_hinten_7_XY" through (-16.25, -16.25, -144) normal (0, 0, 1) x (1, 0, 0)
ref_plane "CP_hinten_7_YZ" through (-16.25, -16.25, -144) normal (1, 0, 0) x (0, 1, 0)
ref_plane "CP_hinten_7_ZX" through (-16.25, -16.25, -144) normal (0, 1, 0) x (0, 0, 1)
ref_plane "CP_hinten_8_XY" through (-16.25, 16.25, -144) normal (0, 0, 1) x (1, 0, 0)
ref_plane "CP_hinten_8_YZ" through (-16.25, 16.25, -144) normal (1, 0, 0) x (0, 1, 0)
ref_plane "CP_hinten_8_ZX" through (-16.25, 16.25, -144) normal (0, 1, 0) x (0, 0, 1)
ref_plane "CP_vorn_1_XY" through (16.25, 16.25, 0) normal (0, 0, 1) x (1, 0, 0)
ref_plane "CP_vorn_1_YZ" through (16.25, 16.25, 0) normal (1, 0, 0) x (0, 1, 0)
ref_plane "CP_vorn_1_ZX" through (16.25, 16.25, 0) normal (0, 1, 0) x (0, 0, 1)
ref_plane "CP_vorn_2_XY" through (16.25, -16.25, 0) normal (0, 0, 1) x (1, 0, 0)
ref_plane "CP_vorn_2_YZ" through (16.25, -16.25, 0) normal (1, 0, 0) x (0, 1, 0)
ref_plane "CP_vorn_2_ZX" through (16.25, -16.25, 0) normal (0, 1, 0) x (0, 0, 1)
ref_plane "CP_vorn_3_XY" through (-16.25, -16.25, 0) normal (0, 0, 1) x (1, 0, 0)
ref_plane "CP_vorn_3_YZ" through (-16.25, -16.25, 0) normal (1, 0, 0) x (0, 1, 0)
ref_plane "CP_vorn_3_ZX" through (-16.25, -16.25, 0) normal (0, 1, 0) x (0, 0, 1)
ref_plane "CP_vorn_4_XY" through (-16.25, 16.25, 0) normal (0, 0, 1) x (1, 0, 0)
ref_plane "CP_vorn_4_YZ" through (-16.25, 16.25, 0) normal (1, 0, 0) x (0, 1, 0)
ref_plane "CP_vorn_4_ZX" through (-16.25, 16.25, 0) normal (0, 1, 0) x (0, 0, 1)
ref_plane "DROSSEL_HINTEN_XY" through (-5.2, 22.75, -128.4) normal (0, 1, 0) x (1, 0, 0)
ref_plane "DROSSEL_HINTEN_YZ" through (-5.2, 22.75, -128.4) normal (1, 0, 0) x (0, 0, -1)
ref_plane "DROSSEL_HINTEN_ZX" through (-5.2, 22.75, -128.4) normal (0, 0, -1) x (0, 1, 0)
ref_plane "DROSSEL_VORN_XY" through (5.2, 22.75, -15.6) normal (0, 1, 0) x (1, 0, 0)
ref_plane "DROSSEL_VORN_YZ" through (5.2, 22.75, -15.6) normal (1, 0, 0) x (0, 0, -1)
ref_plane "DROSSEL_VORN_ZX" through (5.2, 22.75, -15.6) normal (0, 0, -1) x (0, 1, 0)
ref_plane "FDT_SMB_XY" through (0, 22.25, -72) normal (0, 1, 0) x (1, 0, 0)
ref_plane "FDT_SMB_YZ" through (0, 22.25, -72) normal (1, 0, 0) x (0, 0, -1)
ref_plane "FDT_SMB_ZX" through (0, 22.25, -72) normal (0, 0, -1) x (0, 1, 0)
ref_plane "FITTING_1_XY" through (5.2, 22.75, -15.6) normal (0, 1, 0) x (1, 0, 0)
ref_plane "FITTING_1_YZ" through (5.2, 22.75, -15.6) normal (1, 0, 0) x (0, 0, -1)
ref_plane "FITTING_1_ZX" through (5.2, 22.75, -15.6) normal (0, 0, -1) x (0, 1, 0)
ref_plane "FITTING_2_XY" through (-5.2, 22.75, -128.4) normal (0, 1, 0) x (1, 0, 0)
ref_plane "FITTING_2_YZ" through (-5.2, 22.75, -128.4) normal (1, 0, 0) x (0, 0, -1)
ref_plane "FITTING_2_ZX" through (-5.2, 22.75, -128.4) normal (0, 0, -1) x (0, 1, 0)
ref_plane "KOLBEN_XY" through (0, 0, -97) normal (0, 0, 1) x (1, 0, 0)
ref_plane "KOLBEN_YZ" through (0, 0, -97) normal (1, 0, 0) x (0, 1, 0)
ref_plane "KOLBEN_ZX" through (0, 0, -97) normal (0, 1, 0) x (0, 0, 1)
ref_plane "KP_HINTEN_XY" through (0, 0, -144) normal (0, 0, 1) x (1, 0, 0)
ref_plane "KP_HINTEN_YZ" through (0, 0, -144) normal (1, 0, 0) x (0, 1, 0)
ref_plane "KP_HINTEN_ZX" through (0, 0, -144) normal (0, 1, 0) x (0, 0, 1)
ref_plane "KP_VORN_XY" through (0, 0, 0) normal (0, 0, 1) x (1, 0, 0)
ref_plane "KP_VORN_YZ" through (0, 0, 0) normal (1, 0, 0) x (0, 1, 0)
ref_plane "KP_VORN_ZX" through (0, 0, 0) normal (0, 1, 0) x (0, 0, 1)
ref_plane "NUT3_XY" through (-17.75, 6.85, -72) normal (-1, 0, 0) x (0, 1, 0)
ref_plane "NUT3_YZ" through (-17.75, 6.85, -72) normal (0, 1, 0) x (0, 0, -1)
ref_plane "NUT3_ZX" through (-17.75, 6.85, -72) normal (0, 0, -1) x (-1, 0, 0)
ref_plane "NUT4_XY" through (-17.75, -6.85, -72) normal (-1, 0, 0) x (0, 1, 0)
ref_plane "NUT4_YZ" through (-17.75, -6.85, -72) normal (0, 1, 0) x (0, 0, -1)
ref_plane "NUT4_ZX" through (-17.75, -6.85, -72) normal (0, 0, -1) x (-1, 0, 0)
ref_plane "NUT5_XY" through (-6.85, -17.75, -72) normal (0, -1, 0) x (-1, 0, 0)
ref_plane "NUT5_YZ" through (-6.85, -17.75, -72) normal (-1, 0, 0) x (0, 0, -1)
ref_plane "NUT5_ZX" through (-6.85, -17.75, -72) normal (0, 0, -1) x (0, -1, 0)
ref_plane "NUT6_XY" through (6.85, -17.75, -72) normal (0, -1, 0) x (-1, 0, 0)
ref_plane "NUT6_YZ" through (6.85, -17.75, -72) normal (-1, 0, 0) x (0, 0, -1)
ref_plane "NUT6_ZX" through (6.85, -17.75, -72) normal (0, 0, -1) x (0, -1, 0)
ref_plane "NUT7_XY" through (17.75, -6.85, -72) normal (1, 0, 0) x (0, -1, 0)
ref_plane "NUT7_YZ" through (17.75, -6.85, -72) normal (0, -1, 0) x (0, 0, -1)
ref_plane "NUT7_ZX" through (17.75, -6.85, -72) normal (0, 0, -1) x (1, 0, 0)
ref_plane "NUT8_XY" through (17.75, 6.85, -72) normal (1, 0, 0) x (0, -1, 0)
ref_plane "NUT8_YZ" through (17.75, 6.85, -72) normal (0, -1, 0) x (0, 0, -1)
ref_plane "NUT8_ZX" through (17.75, 6.85, -72) normal (0, 0, -1) x (1, 0, 0)
ref_plane "QS_HINTEN_XY" through (-5.2, 22.75, -128.4) normal (0, 1, 0) x (1, 0, 0)
ref_plane "QS_HINTEN_YZ" through (-5.2, 22.75, -128.4) normal (1, 0, 0) x (0, 0, -1)
ref_plane "QS_HINTEN_ZX" through (-5.2, 22.75, -128.4) normal (0, 0, -1) x (0, 1, 0)
ref_plane "QS_VORNE_XY" through (5.2, 22.75, -15.6) normal (0, 1, 0) x (1, 0, 0)
ref_plane "QS_VORNE_YZ" through (5.2, 22.75, -15.6) normal (1, 0, 0) x (0, 0, -1)
ref_plane "QS_VORNE_ZX" through (5.2, 22.75, -15.6) normal (0, 0, -1) x (0, 1, 0)
ref_plane "START_XY" through (0, 0, 0) normal (0, 0, 1) x (1, 0, 0)
ref_plane "START_YZ" through (0, 0, 0) normal (1, 0, 0) x (0, 1, 0)
ref_plane "START_ZX" through (0, 0, 0) normal (0, 1, 0) x (0, 0, 1)
ref_plane "VENTIL_LINKS_XY" through (-24.25, -6.85, -71.9) normal (1, 0, 0) x (0, 0, -1)
ref_plane "VENTIL_LINKS_YZ" through (-24.25, -6.85, -71.9) normal (0, 0, -1) x (0, 1, 0)
ref_plane "VENTIL_LINKS_ZX" through (-24.25, -6.85, -71.9) normal (0, 1, 0) x (1, 0, 0)
ref_plane "VENTIL_RECHTS_XY" through (24.25, -6.85, -71.9) normal (1, 0, 0) x (0, 0, -1)
ref_plane "VENTIL_RECHTS_YZ" through (24.25, -6.85, -71.9) normal (0, 0, -1) x (0, 1, 0)
ref_plane "VENTIL_RECHTS_ZX" through (24.25, -6.85, -71.9) normal (0, 1, 0) x (1, 0, 0)
ref_plane "ZAPFEN_XY" through (0, 0, -40.1) normal (0, 0, 1) x (1, 0, 0)
ref_plane "ZAPFEN_YZ" through (0, 0, -40.1) normal (1, 0, 0) x (0, 1, 0)
ref_plane "ZAPFEN_ZX" through (0, 0, -40.1) normal (0, 1, 0) x (0, 0, 1)
ref_plane "ZUBEHOER_HINTEN_XY" through (0, 0, -144) normal (0, 0, 1) x (1, 0, 0)
ref_plane "ZUBEHOER_HINTEN_YZ" through (0, 0, -144) normal (1, 0, 0) x (0, 1, 0)
ref_plane "ZUBEHOER_HINTEN_ZX" through (0, 0, -144) normal (0, 1, 0) x (0, 0, 1)
ref_plane "ZUBEHOER_VORN_XY" through (0, 0, 0) normal (0, 0, 1) x (1, 0, 0)
ref_plane "ZUBEHOER_VORN_YZ" through (0, 0, 0) normal (1, 0, 0) x (0, 1, 0)
ref_plane "ZUBEHOER_VORN_ZX" through (0, 0, 0) normal (0, 1, 0) x (0, 0, 1)
body "Solid1"
